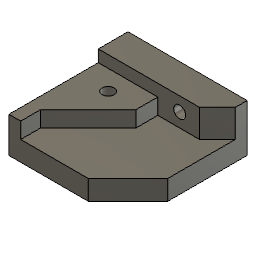
mech task 1 part 1 (Autodesk Fusion 360 design; units mm, degrees)
part number: 2026-03-05-19-05-06-233
Autodesk Fusion 360 part; units mm, degrees
sketch "Sketch1" plane through (0, 0, 0) normal (0, 1, 0) x (1, 0, 0)
  line L0 (0, 0) -> (300, 0)
  line L1 (300, 0) -> (300, 300)
  line L2 (300, 300) -> (0, 300)
  line L3 (0, 300) -> (0, 0)
  line L4 (0, 0) -> (200, 0)
  line L5 (300, 300) -> (300, 100)
  line L6 (200, 0) -> (300, 100)
  dimension "d1" = 300
  dimension "d2" = 300
  dimension "d3" = 200
  dimension "d4" = 200
  constraint horizontal L0
  constraint vertical L1
  constraint horizontal L2
  constraint vertical L3
  constraint coincident L0.start L3.end
  constraint perpendicular L3 L4
  constraint vertical L5
  measures "d1" distance of L0.start L0.end
  measures "d2" distance of L0.start L2.end
  measures "d3" distance of L0.start L4.end
  measures "d4" distance of L1.end L5.end
  measures "d13" angle of L4.end
  measures "d15" angle of L4.end
extrude "Extrude1" add sketch "Sketch1" along normal blind 50 contours L0 L1 L2 L3 L4 L5 L6
sketch "Sketch2" plane through (0, 50, 0) normal (0, 1, 0) x (-1, 0, 0)
  line L0 (-300, -300) -> (0, -300)
  line L1 (0, -300) -> (0, 0)
  line L2 (0, 0) -> (-200, 0)
  line L3 (-200, 0) -> (-300, -100)
  line L4 (-300, -100) -> (-300, -300)
  line L5 (0, 0) -> (-30, 0)
  line L6 (-300, -300) -> (-300, -270)
  line L7 (0, -300) -> (0, -270)
  line L8 (0, -300) -> (0, -240)
  line L9 (-300, -270) -> (-255, -225)
  line L10 (0, -300) -> (0, -225)
  line L11 (0, -225) -> (-255, -225)
  line L12 (-30, 0) -> (-30, -50)
  line L13 (-30, -50) -> (-145.4741, -165.4741)
  line L14 (-30, -50) -> (133.305, -50) construction
  line L15 (0, -225) -> (-150, -225)
  line L16 (-150, -225) -> (-150, -170)
  line L17 (-30, -50) -> (-150, -170)
  line L18 (-30, -50) -> (157.6281, -50) construction
  dimension "d7" = 30
  dimension "d8" = 30
  dimension "d9" = 60
  dimension "d11" = 75
  dimension "d12" = 50
  dimension "d13" = 135
  dimension "d14" = 150
  dimension "d15" = 135
  constraint coincident L1.end L2.start
  constraint perpendicular L1 L5
  constraint coincident L0.start L4.end
  constraint perpendicular L0 L6
  constraint coincident L0.end L1.start
  constraint perpendicular L0 L8
  constraint midpoint L8 L7.end
  constraint vertical L10
  constraint perpendicular L4 L11
  constraint perpendicular L5 L12
  constraint horizontal L14
  constraint perpendicular L1 L15
  constraint perpendicular L11 L16
  constraint horizontal L18
  measures "d7" distance of L1.end L5.end
  measures "d8" distance of L0.start L6.end
  measures "d9" distance of L0.end L8.end
  measures "d11" distance of L0.end L10.end
  measures "d12" distance of L5.end L12.end
  measures "d13" angle of L13 L14
  measures "d14" distance of L10.end L15.end
  measures "d15" angle of L17 L18
extrude "Extrude2" add sketch "Sketch2" along normal blind 40 contours L1 L2 L5 L11 L12 L13 L15 L16 L17
extrude "Extrude3" add sketch "Sketch2" along normal blind 70 contours L0 L1 L4 L6 L7 L8 L9 L10 L11 L15
sketch "Sketch4" plane through (0, 90, 0) normal (0, 1, 0) x (-1, 0, 0)
  line L0 (0, -225) -> (0, 0)
  line L1 (0, 0) -> (-30, 0)
  line L2 (-30, 0) -> (-30, -50)
  line L3 (-30, -50) -> (-150, -170)
  line L4 (-150, -170) -> (-150, -225)
  line L5 (-150, -225) -> (0, -225)
  circle A0 centre (-75, -175) radius 15
  dimension "d20" = 30
  dimension "d21" = 50
  dimension "d22" = 75
  measures "d20" diameter of A0
  measures "d21" distance of L5 A0.centre
  measures "d22" distance of L0 A0.centre
extrude "Extrude4" cut sketch "Sketch4" against normal blind 250 contours A0
sketch "Sketch5" plane through (0, 0, -225) normal (0, 0, 1) x (1, 0, 0)
  line L0 (0, 90) -> (150, 90)
  line L1 (150, 90) -> (150, 50)
  line L2 (150, 50) -> (255, 50)
  line L3 (255, 50) -> (255, 120)
  line L4 (255, 120) -> (0, 120)
  line L5 (0, 120) -> (0, 90)
  circle A0 centre (205, 85) radius 15
  dimension "d25" = 30
  dimension "d26" = 35
  dimension "d27" = 55
  measures "d25" diameter of A0
  measures "d26" distance of L4 A0.centre
  measures "d27" distance of L1 A0.centre
extrude "Extrude5" cut sketch "Sketch5" against normal blind 410 contours A0
